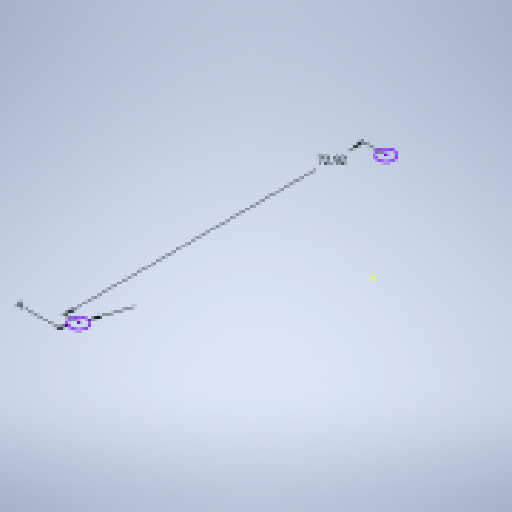
# Autodesk Inventor part: spoolMotorMountPlate
Saved by Autodesk Inventor 2023 (Build 270158000, 158)
## iProperties
Created: 2022-10-11
Part Number: spoolMotorMountPlate
Material: Generic
Document SubType Name: Modeling
Designer: deli
Density: 1 g/cm^3
Appearance: Default
Author: deli
Autodesk Inventor part; units mm, degrees
ref_plane "YZ Plane" through (0, 0, 0) normal (1, 0, 0) x (0, 1, 0)
ref_plane "XZ Plane" through (0, 0, 0) normal (0, 1, 0) x (-1, 0, 0)
ref_plane "XY Plane" through (0, 0, 0) normal (0, 0, 1) x (1, 0, 0)
sketch "Sketch1" plane through (0, 0, 0) normal (0, 1, 0) x (-1, 0, 0)
  circle A0 centre (28.9013, 39.8452) radius 2
  circle A1 centre (28.9013, -33.0748) radius 2
  line L0 (36.9013, -37.0748) -> (24.9013, -37.0748)
  line L1 (24.9013, -37.0748) -> (24.9013, 43.8452)
  line L2 (24.9013, 43.8452) -> (36.9013, 43.8452)
  line L3 (36.9013, 43.8452) -> (36.9013, -37.0748)
  circle A2 centre (32.9013, -12.6148) radius 2
  circle A3 centre (32.9013, 19.3852) radius 2
  point P0 (0, 0)
  dimension "d0" = 4
  dimension "d1" = 72.92
  dimension "d2" = 8
  dimension "d3" = 4
  dimension "d4" = 4
  dimension "d5" = 4
  dimension "d6" = 4
  dimension "d7" = 4
  dimension "d8" = 4
  dimension "d9" = 32
  dimension "d10" = 24.46
  dimension "d11" = 80.92
  constraints: 8 end point, 4 centre point, 3 equal radius, 2 parallel, 1 horizontal, 1 perpendicular
  measures "d0" diameter of A0
  measures "d1" distance of A1.centre A0.centre
  measures "d2" distance from line of L3 A1.centre
  measures "d3" distance from line of L1 A1.centre
  measures "d4" distance from line of L0 A1.centre
  measures "d5" distance from line of L1 A0.centre
  measures "d6" distance from line of L2 A0.centre
  measures "d7" distance from line of L3 A2.centre
  measures "d8" distance from line of L3 A3.centre
  measures "d9" distance of A3.centre A2.centre
  measures "d10" distance from line of L0 A2.centre
  measures "d11" distance of L2.end L0.start
extrude "Extrusion1" add sketch "Sketch1" along normal blind 3.175
equation "\"d4\" = d3"
equation "\"d5\" = d3"
equation "\"d6\" = d4"
equation "\"d7\" = d4"
equation "\"d8\" = d3"
equation "\"d10\" = -0.5 * d9 + 0.5 * d11"
body "Solid1"
